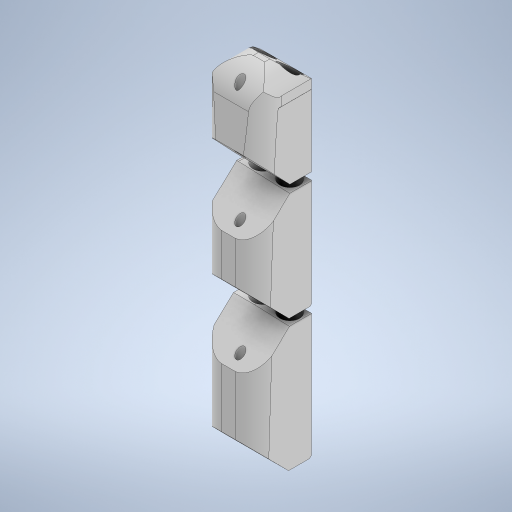
# Autodesk Inventor part: Finger_Index
Saved by Autodesk Inventor 2024 (Build 280153000, 153)
## iProperties
Created: 2025-05-19
Part Number: Finger_Index
Material: Generic
Document SubType Name: Modeling
Designer: Mehdi Charfeddine
Density: 1 g/cm^3
Appearance: Default
Author: Mehdi Charfeddine
Autodesk Inventor part; units mm, degrees
ref_plane "YZ Plane" through (0, 0, 0) normal (1, 0, 0) x (0, 1, 0)
ref_plane "XZ Plane" through (0, 0, 0) normal (0, 1, 0) x (-1, 0, 0)
ref_plane "XY Plane" through (0, 0, 0) normal (0, 0, 1) x (1, 0, 0)
sketch "Sketch1" plane through (0, 0, 0) normal (0, 1, 0) x (-1, 0, 0)
  line L0 (1152.4331, 709.1529) -> (866.3263, 709.1529)
  line L1 (866.3263, 709.1529) -> (855.597, 719.8097)
  line L2 (855.597, 719.8097) -> (855.597, 871.9775)
  line L3 (855.597, 871.9775) -> (850.978, 875.2383)
  line L4 (1152.4331, 709.1529) -> (1163.4823, 719.8097)
  line L5 (1163.4823, 719.8097) -> (1163.4823, 834.5472)
  line L6 (1163.4823, 834.5472) -> (1162.1311, 871.437)
  line L7 (1162.1311, 871.437) -> (1177.2364, 869.2791)
  arc A0 (1162.1311, 871.437) -> (1035.3217, 996.0839) centre (1027.8433, 861.6476) ccw
  line L8 (1035.3217, 996.0839) -> (978.2793, 996.0839)
  line L9 (978.2793, 996.0839) -> (966.9765, 996.0839)
  line L10 (966.9765, 996.0839) -> (962.7973, 1008.4163)
  arc A1 (966.9765, 996.0839) -> (855.597, 871.9775) centre (971.9084, 879.6258) ccw
  arc A2 (1082.7679, 731.2467) -> (1079.7864, 804.7917) centre (1055.8263, 766.9874) ccw
  arc A3 (902.0875, 809.0337) -> (885.0237, 738.7068) centre (918.9713, 767.7035) ccw
  arc A4 (1005.545, 948.5105) -> (969.353, 946.6908) centre (987.3886, 948.8021) ccw
  circle A5 centre (1055.8263, 766.9874) radius 50
  circle A6 centre (918.9713, 767.7035) radius 50
  circle A7 centre (987.3886, 948.8021) radius 20
  point P0 (0, 0)
  dimension "d0" = 100
  dimension "d1" = 100
  dimension "d2" = 40
  constraints: 22 end point, 10 point on circle, 8 centre point, 3 coincident, 2 horizontal, 1 perpendicular, 1 point on line, 1 vertical
  measures "d0" diameter of A5
  measures "d1" diameter of A6
  measures "d2" diameter of A7
extrude "Extrusion1" add sketch "Sketch1" along normal blind 3000
sketch "Sketch2" plane through (0, 0, 0) normal (0, 0, 1) x (1, 0, 0)
  line L0 (-1163.9753, 1042.7115) -> (-866.3356, 1037.0824)
  line L1 (-866.3356, 1037.0824) -> (-860.2374, 1675.0494)
  line L2 (-860.2374, 1675.0494) -> (-1146.6273, 1680.4657)
  line L3 (-1146.6273, 1680.4657) -> (-1163.9753, 1042.7115)
  line L4 (-1147.1024, 1711.9817) -> (-863.7615, 1706.623)
  line L5 (-863.7615, 1706.623) -> (-858.478, 2259.3584)
  line L6 (-858.478, 2259.3584) -> (-1132.0721, 2264.5327)
  line L7 (-1132.0721, 2264.5327) -> (-1147.1024, 1711.9817)
  line L8 (-1131.0467, 2302.2281) -> (-859.2201, 2297.6085)
  line L9 (-859.2201, 2297.6085) -> (-855.7268, 2663.0679)
  line L10 (-855.7268, 2663.0679) -> (-1121.0349, 2670.2847)
  line L11 (-1121.0349, 2670.2847) -> (-1131.0467, 2302.2281)
  arc A0 (-1015.1555, 2799.8873) -> (-1121.0349, 2670.2847) centre (-1014.4692, 2691.276) ccw
  arc A1 (-855.7268, 2663.0679) -> (-957.431, 2799.8873) centre (-966.1453, 2687.1991) ccw
  line L12 (-957.431, 2799.8873) -> (-1015.1555, 2799.8873)
  line L13 (-1499.2309, -337.2841) -> (-196.6788, -337.2841)
  line L14 (-196.6788, -337.2841) -> (-196.6788, 3240.483)
  line L15 (-196.6788, 3240.483) -> (-1499.2309, 3240.483)
  line L16 (-1499.2309, 3240.483) -> (-1499.2309, -337.2841)
  point P0 (0, 0)
  constraints: 34 end point, 8 parallel, 4 point on circle, 3 perpendicular, 2 centre point, 2 horizontal, 1 point on line
extrude "Extrusion2" cut sketch "Sketch2" along normal mid plane 3000
sketch "Sketch3" plane through (0, 0, 0) normal (1, 0, 0) x (0, 1, 0)
  line L0 (404.2545, 1541.1016) -> (3429.5205, 1541.1016)
  line L1 (3429.5205, 1541.1016) -> (3429.5205, 87.3038)
  line L2 (3429.5205, 87.3038) -> (404.2545, 87.3038)
  line L3 (404.2545, 87.3038) -> (404.2545, 1541.1016)
  line L4 (1037.693, 825.9608) -> (1037.693, 719.6095)
  line L5 (1037.693, 719.6095) -> (1048.5475, 709.0513)
  line L6 (1048.5475, 709.0513) -> (1669.7199, 709.0513)
  line L7 (1669.7199, 709.0513) -> (1678.4571, 718.0336)
  line L8 (1678.4571, 718.0336) -> (1678.4571, 824.3848)
  line L9 (1678.4571, 824.3848) -> (1508.153, 996.2653)
  line L10 (1508.153, 996.2653) -> (1209.5741, 996.2653)
  line L11 (1209.5741, 996.2653) -> (1037.693, 825.9608)
  line L12 (1706.6572, 825.8812) -> (1706.6572, 719.5299)
  line L13 (1706.6572, 719.5299) -> (1717.0398, 709.0513)
  line L14 (1717.0398, 709.0513) -> (2253.7727, 709.0513)
  line L15 (2253.7727, 709.0513) -> (2264.3668, 719.5482)
  line L16 (2264.3668, 719.5482) -> (2264.3668, 822.6428)
  line L17 (2264.3668, 822.6428) -> (2092.3368, 996.2653)
  line L18 (2092.3368, 996.2653) -> (1878.6187, 996.2653)
  line L19 (1878.6187, 996.2653) -> (1706.6572, 825.8812)
  line L20 (2296.8101, 825.6603) -> (2296.8101, 719.539)
  line L21 (2296.8101, 719.539) -> (2307.2016, 709.0513)
  line L22 (2307.2016, 709.0513) -> (2699.8876, 709.0513)
  line L23 (2699.8876, 709.0513) -> (2800.042, 829.387)
  line L24 (2800.042, 829.387) -> (2800.042, 853.9846)
  line L25 (2800.042, 853.9846) -> (2821.6104, 859.0737)
  line L26 (2296.8101, 825.6603) -> (2468.9231, 989.2012)
  line L27 (2468.9231, 989.2012) -> (2665.8515, 980.7518)
  line L28 (2665.8515, 980.7518) -> (2669.9138, 992.9387)
  arc A0 (2800.042, 853.9846) -> (2665.8515, 980.7518) centre (2659.8102, 839.9488) ccw
  point P0 (0, 0)
  constraints: 58 end point, 8 parallel, 7 perpendicular, 6 point on line, 3 vertical, 2 point on circle, 1 centre point, 1 horizontal, 1 tangent
extrude "Extrusion3" cut sketch "Sketch3" along normal mid plane 3000
sketch "Sketch4" plane through (-866.3263, 1716.9391, 709.1529) normal (0, 0, -1) x (-1, 0, 0)
  line L0 (256.4077, 983.033) -> (0, 983.033) projected
  line L1 (264.5878, 590.1618) -> (264.7204, 585.289) projected
  line L2 (0, 983.033) -> (264.5878, 590.1618)
  line L3 (264.5878, 590.1618) -> (0.0242, 587.6329)
  line L4 (-7.9088, 664.641) -> (-7.1062, 580.6694) projected
  line L5 (0.0242, 587.6329) -> (253.8096, 983.033)
  line L6 (0, 0) -> (280.6412, 0) projected
  line L7 (0.5199, 535.7723) -> (280.6412, 0)
  line L8 (280.6412, 0) -> (264.5878, 535.7723)
  line L9 (264.5878, 535.7723) -> (0, 0)
  line L10 (0, -47.1203) -> (-5.4268, -41.8772) projected
  line L11 (286.1069, -668.4961) -> (286.1069, -249.9092) projected
  line L12 (0, -47.1203) -> (286.1069, -668.4961)
  line L13 (286.1069, -668.4961) -> (282.0514, -47.0645)
  line L14 (0, -668.4961) -> (286.1069, -668.4961) projected
  line L15 (282.0514, -47.0645) -> (0, -668.4961)
  line L16 (111.3191, 251.0368) -> (161.3191, 251.0368)
  line L17 (161.3191, 251.0368) -> (161.3191, 301.0368)
  line L18 (161.3191, 301.0368) -> (111.3191, 301.0368)
  line L19 (111.3191, 301.0368) -> (111.3191, 251.0368)
  line L20 (111.3191, 251.0368) -> (161.3191, 301.0368) construction
  line L21 (161.3191, 251.0368) -> (111.3191, 301.0368) construction
  line L22 (117.0259, -380.5766) -> (167.0259, -380.5766)
  line L23 (167.0259, -380.5766) -> (167.0259, -330.5766)
  line L24 (167.0259, -330.5766) -> (117.0259, -330.5766)
  line L25 (117.0259, -330.5766) -> (117.0259, -380.5766)
  line L26 (117.0259, -380.5766) -> (167.0259, -330.5766) construction
  line L27 (167.0259, -380.5766) -> (117.0259, -330.5766) construction
  line L28 (104.9563, 765.0684) -> (154.9563, 765.0684)
  line L29 (154.9563, 765.0684) -> (154.9563, 815.0684)
  line L30 (154.9563, 815.0684) -> (104.9563, 815.0684)
  line L31 (104.9563, 815.0684) -> (104.9563, 765.0684)
  line L32 (104.9563, 765.0684) -> (154.9563, 815.0684) construction
  line L33 (154.9563, 765.0684) -> (104.9563, 815.0684) construction
  line L34 (154.9563, 815.0684) -> (204.9563, 815.0684)
  line L35 (204.9563, 815.0684) -> (204.9563, 765.0684)
  line L36 (204.9563, 765.0684) -> (154.9563, 765.0684)
  line L37 (154.9563, 765.0684) -> (154.9563, 815.0684)
  arc A0 (204.9563, 765.0684) -> (154.9563, 815.0684) centre (154.9563, 765.0684) ccw
  line L38 (104.9563, 815.0684) -> (54.9563, 815.0684)
  line L39 (54.9563, 815.0684) -> (54.9563, 865.0684)
  line L40 (54.9563, 865.0684) -> (104.9563, 865.0684)
  line L41 (104.9563, 865.0684) -> (104.9563, 815.0684)
  line L42 (104.9563, 765.0684) -> (54.9563, 765.0684)
  line L43 (54.9563, 765.0684) -> (54.9563, 665.0684)
  line L44 (54.9563, 665.0684) -> (104.9563, 665.0684)
  line L45 (104.9563, 665.0684) -> (104.9563, 765.0684)
  line L46 (154.9563, 765.0684) -> (204.9563, 765.0684)
  line L47 (204.9563, 765.0684) -> (204.9563, 665.0684)
  line L48 (204.9563, 665.0684) -> (154.9563, 665.0684)
  line L49 (154.9563, 665.0684) -> (154.9563, 765.0684)
  line L50 (111.3191, 301.0368) -> (61.3191, 301.0368)
  line L51 (61.3191, 301.0368) -> (61.3191, 351.0368)
  line L52 (61.3191, 351.0368) -> (111.3191, 351.0368)
  line L53 (111.3191, 351.0368) -> (111.3191, 301.0368)
  line L54 (111.3191, 251.0368) -> (61.3191, 251.0368)
  line L55 (61.3191, 251.0368) -> (61.3191, 151.0368)
  line L56 (61.3191, 151.0368) -> (111.3191, 151.0368)
  line L57 (111.3191, 151.0368) -> (111.3191, 251.0368)
  line L58 (61.3191, 251.0368) -> (111.3191, 251.0368)
  line L59 (111.3191, 251.0368) -> (111.3191, 301.0368)
  line L60 (111.3191, 301.0368) -> (61.3191, 301.0368)
  line L61 (61.3191, 301.0368) -> (61.3191, 251.0368)
  arc A1 (61.3191, 201.0368) -> (111.3191, 151.0368) centre (111.3191, 201.0368) ccw
  line L62 (111.3191, 151.0368) -> (161.3191, 151.0368)
  line L63 (161.3191, 151.0368) -> (161.3191, 201.0368)
  line L64 (161.3191, 201.0368) -> (111.3191, 201.0368)
  line L65 (111.3191, 201.0368) -> (111.3191, 151.0368)
  line L66 (117.0259, -380.5766) -> (167.0259, -380.5766)
  line L67 (167.0259, -380.5766) -> (167.0259, -480.5766)
  line L68 (167.0259, -480.5766) -> (117.0259, -480.5766)
  line L69 (117.0259, -480.5766) -> (117.0259, -380.5766)
  line L70 (117.0259, -480.5766) -> (17.0259, -480.5766)
  line L71 (17.0259, -480.5766) -> (17.0259, -430.5766)
  line L72 (17.0259, -430.5766) -> (117.0259, -430.5766)
  line L73 (117.0259, -430.5766) -> (117.0259, -480.5766)
  line L74 (17.0259, -430.5766) -> (67.0259, -430.5766)
  line L75 (67.0259, -430.5766) -> (67.0259, -330.5766)
  line L76 (67.0259, -330.5766) -> (17.0259, -330.5766)
  line L77 (17.0259, -330.5766) -> (17.0259, -430.5766)
  line L78 (167.0259, -480.5766) -> (217.0259, -480.5766)
  line L79 (217.0259, -480.5766) -> (217.0259, -430.5766)
  line L80 (217.0259, -430.5766) -> (167.0259, -430.5766)
  line L81 (167.0259, -430.5766) -> (167.0259, -480.5766)
  line L82 (217.0259, -430.5766) -> (267.0259, -430.5766)
  line L83 (267.0259, -430.5766) -> (267.0259, -330.5766)
  line L84 (267.0259, -330.5766) -> (217.0259, -330.5766)
  line L85 (217.0259, -330.5766) -> (217.0259, -430.5766)
  arc A2 (17.0259, -430.5766) -> (67.0259, -480.5766) centre (67.0259, -430.5766) ccw
  point P0 (-866.3263, -1716.9391)
  point P1 (136.3191, 276.0368)
  point P2 (142.0259, -355.5766)
  point P3 (129.9563, 790.0684)
  point P4 (167.0259, -430.5766)
  point P5 (167.0259, -380.5766)
  point P6 (117.0259, -430.5766)
  point P7 (67.0259, -430.5766)
  point P8 (61.3191, 301.0368)
  point P9 (111.3191, 201.0368)
  point P10 (154.9563, 765.0684)
  point P11 (204.9563, 765.0684)
  dimension "d9" = 50
  dimension "d10" = 50
  dimension "d11" = 50
  dimension "d12" = 50
  dimension "d13" = 50
  dimension "d14" = 50
  dimension "d15" = 50
  dimension "d16" = 50
  dimension "d17" = 50
  dimension "d18" = 50
  dimension "d19" = 50
  dimension "d20" = 100
  dimension "d21" = 50
  dimension "d22" = 50
  dimension "d23" = 50
  dimension "d24" = 100
  dimension "d25" = 50
  dimension "d26" = 50
  dimension "d27" = 50
  dimension "d28" = 50
  dimension "d29" = 100
  dimension "d30" = 100
  dimension "d31" = 50
  dimension "d32" = 50
  dimension "d33" = 50
  dimension "d34" = 50
  dimension "d35" = 100
  dimension "d36" = 50
  constraints: 158 end point, 32 parallel, 17 perpendicular, 16 horizontal, 8 midpoint, 7 point on line, 6 point on circle, 3 centre point
  measures "d9" distance of L18.end L17.end
  measures "d10" distance of L17.end L16.end
  measures "d11" distance of L24.end L23.end
  measures "d12" distance of L23.end L22.end
  measures "d13" distance of L30.end L29.end
  measures "d14" distance of L29.end L28.end
  measures "d15" distance of L35.end L36.end
  measures "d16" radius of A0
  measures "d17" distance of L39.end L40.end
  measures "d18" distance of L38.end L39.end
  measures "d19" distance of L44.end L43.end
  measures "d20" distance of L43.end L42.end
  measures "d21" distance of L51.end L52.end
  measures "d22" distance of L50.end L51.end
  measures "d23" distance of L56.end L55.end
  measures "d24" distance of L55.end L54.end
  measures "d25" radius of A1
  measures "d26" distance of L64.end L63.end
  measures "d27" distance of L63.end L62.end
  measures "d28" distance of L67.end L68.end
  measures "d29" distance of L66.end L67.end
  measures "d30" distance of L71.end L72.end
  measures "d31" distance of L70.end L71.end
  measures "d32" distance of L80.end L79.end
  measures "d33" distance of L79.end L78.end
  measures "d34" distance of L84.end L83.end
  measures "d35" distance of L83.end L82.end
  measures "d36" radius of A2
extrude "Extrusion4" add sketch "Sketch4" along normal blind 10 contours L30 L29 L28 L2 L5 | L5 L2 L30 | L40 L41 L2 | L2 L41 L38 L39 L40 | L5 L28 L31 L30 L2 | L2 L28 L5 | A0 L36 L29 | L36 L47 L2 L49 | L2 L47 L48 L49 | L45 L44 L43 L5 | L5 L43 L42 L45 | L16 L9 L7 | L7 L9 L18 L17 L16 | A1 L55 L54 L57 L9 | L9 L57 A1 | L57 L64 L63 L62 | L9 L16 L19 L18 L7 | L7 L18 L9 | L54 L61 L50 L19 | L53 L50 L51 L52 L7 | L7 L52 L53 | L24 L15 L12 | L12 L15 L22 L25 L24 | L15 L24 L23 L22 L12 | L12 L22 L15 | L85 L84 L83 L82 | L22 L67 L12 | L12 L67 L68 L69 L15 L22 | L15 L69 L22 | L80 L79 L78 L12 | L12 L78 L67 L80 | L72 L69 L70 L15 | L15 L70 A2 L72 | L72 L77 L76 L75
body "Solid1"
